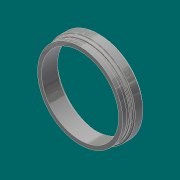
# Autodesk Inventor part: A1-19027-100-xx 32in Type B victaulic ring
Saved by Autodesk Inventor 2017.3 (Build 213256000, 256)
## iProperties
Created: 2013-12-16
Part Number: A1-19027-100-xx 32in Type B victaulic ring
Material: Steel, Mild
Document SubType Name: Modeling
Designer: Graeme_Van_Dongen
Density: 7.86 g/cm^3
Appearance: Steel
Description: 32" TYPE B VICTAULIC RING FOR STYLE 275 COUPLING, A105N, CUSTOM INVERTED B
Mass: 173717 g
Surface Area: 14137 cm^2
Volume: 22101.4 cm^3
Author: Graeme_Van_Dongen
Autodesk Inventor part; units mm, degrees
ref_plane "YZ Plane" through (0, 0, 0) normal (1, 0, 0) x (0, 1, 0)
ref_plane "XZ Plane" through (0, 0, 0) normal (0, 1, 0) x (-1, 0, 0)
ref_plane "XY Plane" through (0, 0, 0) normal (0, 0, 1) x (1, 0, 0)
sketch "Sketch1" plane through (0, 0, 0) normal (1, 0, 0) x (0, 1, 0)
  line L0 (396.875, 0) -> (396.875, 165.1)
  line L1 (396.875, 165.1) -> (438.15, 165.1)
  line L2 (438.15, 165.1) -> (438.15, 122.322)
  line L3 (438.15, 122.322) -> (425.45, 120.65)
  line L4 (425.45, 120.65) -> (425.45, 86.36)
  line L5 (425.45, 86.36) -> (438.15, 83.6026)
  line L6 (438.15, 83.6026) -> (438.15, 73.66)
  line L7 (0, -78.74) -> (0, 205.74) projected
  arc A0 (438.15, 73.66) -> (444.5, 62.6615) centre (450.85, 73.66) ccw
  line L8 (444.5, 62.6615) -> (457.2, 55.3291)
  line L9 (457.2, 55.3291) -> (457.2, -23.2231)
  line L10 (457.2, -23.2231) -> (446.0875, -31.75)
  line L11 (446.0875, -31.75) -> (441.325, -31.75)
  line L12 (441.325, -31.75) -> (441.325, -38.1)
  line L13 (441.325, -38.1) -> (439.7375, -38.1)
  line L14 (439.7375, -38.1) -> (439.7375, -12.7)
  arc A1 (439.7375, -12.7) -> (427.0375, 0) centre (427.0375, -12.7) ccw
  line L15 (427.0375, 0) -> (396.875, 0)
  point P0 (0, 0)
  dimension "d0" = 396.875
  dimension "d5" = 165.1
  dimension "d13" = 425.45
  dimension "d14" = 438.15
  dimension "d16" = 44.45
  dimension "d17" = 34.29
  dimension "d18" = 7.5
  dimension "d19" = 12.25
  dimension "d32" = 457.2
  dimension "d33" = 11.1125
  dimension "d34" = 4.7625
  dimension "d35" = 1.5875
  dimension "d36" = 12.7
  dimension "d37" = 37.5
  dimension "d38" = 203.2
  dimension "d39" = 6.35
  dimension "d40" = 12.7
  dimension "d41" = 30
  dimension "d42" = 12.7
  constraints: 30 end point, 6 perpendicular, 4 point on circle, 4 tangent, 3 parallel, 2 centre point, 2 vertical, 1 collinear, 1 point on line
  measures "d0" distance from line of point (0, 0) L0
  measures "d5" distance of L0.start L0.end
  measures "d13" distance from line of point (0, 0) L4
  measures "d14" distance from line of point (0, 0) L6
  measures "d16" distance from line of L3.end L1
  measures "d17" distance of L3.end L4.end
  measures "d18" angle of L1 L3
  measures "d19" angle of L5 L1
  measures "d32" distance between parallel lines of L7 L9
  measures "d33" horizontal distance of L9.end L10.end
  measures "d34" distance of L10.end L11.end
  measures "d35" distance of L12.end L13.end
  measures "d36" radius of A1
  measures "d37" angle of L11 L10
  measures "d38" distance between parallel lines of L13 L1
  measures "d39" distance of L11.end L12.end
  measures "d40" radius of A0
  measures "d41" angle of L1 L8
  measures "d42" vertical distance of L4.end A0.centre
revolve "Revolution1" add sketch "Sketch1" angle 360 about axis through (0, 0, -10) along (0, 0, 1)
chamfer "Chamfer2" distance 0.7937 angle 45 1 edges at (0, -396.875, 0)
body "Solid1"
